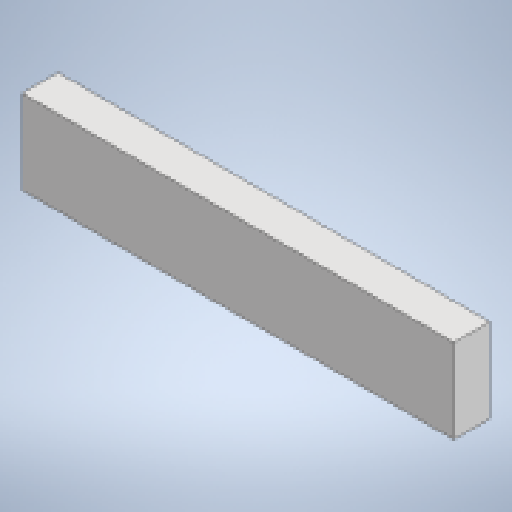
# Autodesk Inventor part: back-side
Saved by Autodesk Inventor 2025.1 (Build 291241020, 241B)
## iProperties
Created: 2024-09-20
Part Number: back-side
Material: Generic
Document SubType Name: Modeling
Designer: User
Density: 1 g/cm^3
Appearance: Default
Author: User
Autodesk Inventor part; units mm, degrees
ref_plane "YZ Plane" through (0, 0, 0) normal (1, 0, 0) x (0, 1, 0)
ref_plane "XZ Plane" through (0, 0, 0) normal (0, 1, 0) x (-1, 0, 0)
ref_plane "XY Plane" through (0, 0, 0) normal (0, 0, 1) x (1, 0, 0)
sketch "Sketch1" plane through (0, 0, 0) normal (0, 0, 1) x (1, 0, 0)
  line L0 (0, 1219.2) -> (0, 0) projected
  line L1 (-457.2, 0) -> (-457.2, 1219.2) projected
  line L2 (0, 0) -> (-457.2, 0)
  line L3 (-457.2, 88.9) -> (0, 88.9)
  dimension "d0" = 88.9
  constraints: 4 end point, 2 perpendicular, 2 point on line
  measures "d0" distance between parallel lines of L3 L2
extrude "Extrusion1" add sketch "Sketch1" against normal blind 38.1
body "Solid1"
